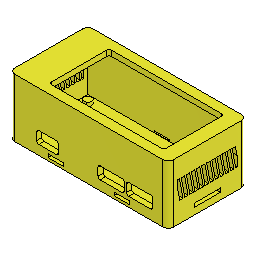
cubiea7z (Autodesk Fusion 360 design; units mm, degrees)
part number: 2026-06-29-06-27-47-318
Autodesk Fusion 360 part; units mm, degrees
sketch "Sketch1" plane through (0, 0, 0) normal (0, 0, 1) x (1, 0, 0)
  line L0 (0, 0) -> (67.4, 0)
  line L1 (67.4, 0) -> (67.4, -30.75)
  line L2 (67.4, -30.75) -> (0, -30.75)
  line L3 (0, -30.75) -> (0, 0)
  line L4 (69.9, -33.25) -> (-2.5, -33.25)
  line L5 (-2.5, -33.25) -> (-2.5, 2.5)
  line L6 (-2.5, 2.5) -> (69.9, 2.5)
  line L7 (69.9, 2.5) -> (69.9, -33.25)
  dimension "d1" = 30.75
  dimension "d2" = 67.4
  dimension "d3" = -2.5
  constraint horizontal L0
  constraint vertical L1
  constraint horizontal L2
  constraint vertical L3
  constraint coincident L0.start L3.end
  measures "d1" distance of L0.start L2.end
  measures "d2" distance of L0.start L0.end
extrude "Extrude1" add sketch "Sketch1" against normal blind 2.5 contours L0 L1 L2 L3 | L4 L5 L6 L7 makes body 1
sketch "Sketch2" plane through (0, 0, 0) normal (0, 0, 1) x (1, 0, 0)
  line L0 (67.4, -30.75) -> (0, -30.75)
  line L1 (67.4, 0) -> (67.4, -30.75)
  line L2 (0, 0) -> (67.4, 0)
  line L3 (67.4, -30.75) -> (65.4, -30.75)
  line L4 (65.4, -30.75) -> (65.4, -23.75)
  line L5 (65.4, -23.75) -> (67.4, -23.75)
  line L6 (67.4, -23.75) -> (67.4, -30.75)
  line L7 (67.4, 0) -> (65.4, 0)
  line L8 (65.4, 0) -> (65.4, -5)
  line L9 (65.4, -5) -> (67.4, -5)
  line L10 (67.4, -5) -> (67.4, 0)
  line L11 (0, -30.75) -> (0, 0)
  line L12 (0, 0) -> (2, 0)
  line L13 (2, 0) -> (2, -30.75)
  line L14 (2, -30.75) -> (0, -30.75)
  line L15 (0, -30.75) -> (0, 0)
  line L16 (67.4, 0) -> (63.4, 0)
  line L17 (63.4, 0) -> (63.4, -5)
  line L18 (63.4, -5) -> (67.4, -5)
  line L19 (67.4, -5) -> (67.4, 0)
  line L20 (67.4, -30.75) -> (63.4, -30.75)
  line L21 (63.4, -30.75) -> (63.4, -23.75)
  line L22 (63.4, -23.75) -> (67.4, -23.75)
  line L23 (67.4, -23.75) -> (67.4, -30.75)
  dimension "d6" = 2
  dimension "d7" = 7
  dimension "d8" = 2
  dimension "d9" = 5
  dimension "d10" = 2
  dimension "d11" = 4
  dimension "d12" = 5
  dimension "d13" = 4
  dimension "d14" = 7
  constraint horizontal L3
  constraint vertical L4
  constraint horizontal L5
  constraint vertical L6
  constraint coincident L0.start L1.end
  constraint horizontal L7
  constraint vertical L8
  constraint horizontal L9
  constraint vertical L10
  constraint coincident L1.start L2.end
  constraint horizontal L12
  constraint vertical L13
  constraint horizontal L14
  constraint vertical L15
  constraint coincident L2.start L11.end
  constraint horizontal L16
  constraint vertical L17
  constraint horizontal L18
  constraint vertical L19
  constraint horizontal L20
  constraint vertical L21
  constraint horizontal L22
  constraint vertical L23
  measures "d6" distance of L0.start L3.end
  measures "d7" distance of L0.start L5.end
  measures "d8" distance of L1.start L7.end
  measures "d9" distance of L1.start L9.end
  measures "d10" distance of L2.start L12.end
  measures "d11" distance of L1.start L16.end
  measures "d12" distance of L1.start L9.end
  measures "d13" distance of L0.start L20.end
  measures "d14" distance of L0.start L5.end
extrude "Extrude2" add sketch "Sketch2" along normal blind 1.2 contours L0 L4 L20 L21 L22 | L0 L2 L11 L12 L13 L14 L15 | L2 L8 L16 L17 L18 bodies 1
extrude "Extrude3" add sketch "Sketch2" along normal blind 3 contours L0 L1 L3 L4 L5 L6 L20 L22 L23 | L1 L2 L7 L8 L9 L10 L16 L18 L19 bodies 1
extrude "Extrude4" add sketch "Sketch1" along normal blind 24.1 bodies 1
ref_plane "WorkPlane1" through (34.7, -15.375, 19.4) normal (0, 0, 1) x (1, 0, 0)
sketch "USB-HDMI" plane through (0, -33.25, 0) normal (0, -1, 0) x (1, 0, 0)
  line L0 (-2.5, 24.1) -> (-2.5, -2.5)
  line L1 (-2.5, -2.5) -> (69.9, -2.5)
  line L2 (69.9, -2.5) -> (69.9, 24.1)
  line L3 (69.9, 24.1) -> (-2.5, 24.1)
  line L4 (67.4, 0) -> (63.4, 0)
  line L5 (63.4, 0) -> (2, 0)
  line L6 (2, 0) -> (63.4, 0)
  line L7 (63.4, 0) -> (67.4, 0)
  line L8 (0, 1.2) -> (0, 24.1)
  line L9 (0, 24.1) -> (0, 1.2)
  line L10 (67.4, 3) -> (67.4, 0)
  line L11 (67.4, 0) -> (67.4, 3)
  line L12 (67.4, 3) -> (67.4, 24.1)
  line L13 (67.4, 24.1) -> (67.4, 3)
  line L14 (5, 0) -> (5, 17) construction
  line L15 (5, 17) -> (29, 17) construction
  line L16 (29.5, 14.25) -> (4.5, 14.25)
  line L17 (4.5, 14.25) -> (4.5, 19.75)
  line L18 (4.5, 19.75) -> (29.5, 19.75)
  line L19 (29.5, 19.75) -> (29.5, 14.25)
  line L20 (29.5, 14.25) -> (4.5, 19.75) construction
  line L21 (4.5, 14.25) -> (29.5, 19.75) construction
  line L22 (5, 17) -> (48, 17) construction
  line L23 (48, 17) -> (57, 17) construction
  line L24 (57.5, 14.25) -> (47.5, 14.25)
  line L25 (47.5, 14.25) -> (47.5, 19.75)
  line L26 (47.5, 19.75) -> (57.5, 19.75)
  line L27 (57.5, 19.75) -> (57.5, 14.25)
  line L28 (57.5, 14.25) -> (47.5, 19.75) construction
  line L29 (47.5, 14.25) -> (57.5, 19.75) construction
  line L30 (17, 19.75) -> (17, 14.25) construction
  line L31 (17.5, 14.25) -> (16.5, 14.25)
  line L32 (16.5, 14.25) -> (16.5, 19.75)
  line L33 (16.5, 19.75) -> (17.5, 19.75)
  line L34 (17.5, 19.75) -> (17.5, 14.25)
  line L35 (17.5, 14.25) -> (16.5, 19.75) construction
  line L36 (16.5, 14.25) -> (17.5, 19.75) construction
  point P0 (17, 17)
  point P1 (52.5, 17)
  point P2 (17, 17)
  dimension "d21" = 17
  dimension "d22" = 5
  dimension "d23" = 24
  dimension "d24" = 5.5
  dimension "d25" = 25
  dimension "d26" = 43
  dimension "d27" = 9
  dimension "d28" = 10
  dimension "d29" = 5.5
  dimension "d34" = 1
  constraint perpendicular L6 L14
  constraint perpendicular L14 L15
  constraint horizontal L16
  constraint perpendicular L16 L17
  constraint parallel L16 L18
  constraint parallel L17 L19
  constraint coincident L20 P2
  constraint coincident L21 P2
  constraint midpoint L15 P2
  constraint perpendicular L14 L22
  constraint parallel L22 L23
  constraint horizontal L24
  constraint perpendicular L24 L25
  constraint parallel L24 L26
  constraint parallel L25 L27
  constraint coincident L28 P1
  constraint coincident L29 P1
  constraint midpoint L23 P1
  constraint midpoint L18 L30.start
  constraint midpoint L16 L30.end
  constraint horizontal L31
  constraint perpendicular L31 L32
  constraint parallel L31 L33
  constraint parallel L32 L34
  constraint coincident L35 P2
  constraint coincident L36 P2
  constraint coincident P2 P0
  measures "d21" distance of L14.start L14.end
  measures "d22" distance of L9 L14
  measures "d23" distance of L14.end L15.end
  measures "d24" distance of L16.end L17.end
  measures "d25" distance of L16.start L16.end
  measures "d26" distance of L14.end L22.end
  measures "d27" distance of L22.end L23.end
  measures "d28" distance of L25.end L26.end
  measures "d29" distance of L24.end L25.end
  measures "d34" distance of L32.end L33.end
extrude "Extrude5" cut sketch "USB-HDMI" against normal blind 2.5 contours L16 L18 L19 L34 | L16 L17 L18 L32 | L24 L25 L26 L27 bodies 1
fillet "Fillet1" radius 1 8 edges at (4.5, -32, 19.75) (4.5, -32, 14.25) (29.5, -32, 19.75) (29.5, -32, 14.25) (57.5, -32, 14.25) (57.5, -32, 19.75) (47.5, -32, 19.75) (47.5, -32, 14.25) on bodies 1
fillet "Fillet2" radius 1 4 edges at (17.5, -32, 19.75) (17.5, -32, 14.25) (16.5, -32, 19.75) (16.5, -32, 14.25) on bodies 1
sketch "SD-Cam" plane through (-2.5, 0, 0) normal (-1, 0, 0) x (0, -1, 0)
  line L0 (-2.5, 24.1) -> (-2.5, -2.5)
  line L1 (-2.5, -2.5) -> (33.25, -2.5)
  line L2 (33.25, -2.5) -> (33.25, 24.1)
  line L3 (33.25, 24.1) -> (-2.5, 24.1)
  line L4 (-3.075, 19.4) -> (33.825, 19.4)
  line L5 (15.375, 19.4) -> (9.375, 19.4)
  line L6 (9.375, 19.4) -> (9.375, 21.05)
  line L7 (9.375, 21.05) -> (15.375, 21.05)
  line L8 (15.375, 21.05) -> (15.375, 19.4)
  line L9 (15.375, 19.4) -> (21.375, 19.4)
  line L10 (21.375, 19.4) -> (21.375, 21.05)
  line L11 (21.375, 21.05) -> (15.375, 21.05)
  line L12 (15.375, 21.05) -> (15.375, 19.4)
  dimension "d38" = 6
  dimension "d39" = 1.65
  dimension "d40" = 1.65
  constraint horizontal L5
  constraint vertical L6
  constraint horizontal L7
  constraint vertical L8
  constraint midpoint L4 L5.start
  constraint horizontal L9
  constraint vertical L10
  constraint horizontal L11
  constraint vertical L12
  measures "d38" distance of L5.start L5.end
  measures "d39" distance of L5.start L7.end
  measures "d40" distance of L5.start L7.end
extrude "Extrude6" cut sketch "SD-Cam" against normal blind 2.5 contours L4 L5 L6 L7 L8 L12 | L4 L8 L9 L10 L11 L12 bodies 1
fillet "Fillet3" radius 0.3 4 edges at (-1.25, -9.375, 21.05) (-1.25, -9.375, 19.4) (-1.25, -21.375, 21.05) (-1.25, -21.375, 19.4) on bodies 1
extrude "Extrude7" cut sketch "SD-Cam" against normal blind 72.4 contours L4 L5 L6 L7 L8 L12 | L4 L8 L9 L10 L11 L12 bodies 1
sketch "Antenne" plane through (69.9, 0, 0) normal (1, 0, 0) x (0, 1, 0)
  line L0 (-21.375, 19.4) -> (-21.375, 21.05)
  line L1 (-21.375, 21.05) -> (-9.375, 21.05)
  line L2 (-9.375, 21.05) -> (-9.375, 19.4)
  line L3 (-9.375, 19.4) -> (-21.375, 19.4)
  line L4 (-33.25, 24.1) -> (-33.25, -2.5)
  line L5 (-33.25, -2.5) -> (2.5, -2.5)
  line L6 (2.5, -2.5) -> (2.5, 24.1)
  line L7 (2.5, 24.1) -> (-33.25, 24.1)
  line L8 (3.075, 19.4) -> (-33.825, 19.4)
  line L9 (3.075, 18.4) -> (-33.825, 18.4) construction
  line L10 (-15.375, 18.4) -> (-17.375, 18.4)
  line L11 (-17.375, 18.4) -> (-17.375, 15.4)
  line L12 (-17.375, 15.4) -> (-15.375, 15.4)
  line L13 (-15.375, 15.4) -> (-15.375, 18.4)
  line L14 (-15.375, 18.4) -> (-13.375, 18.4)
  line L15 (-13.375, 18.4) -> (-13.375, 15.4)
  line L16 (-13.375, 15.4) -> (-15.375, 15.4)
  line L17 (-15.375, 15.4) -> (-15.375, 18.4)
  dimension "d47" = -1
  dimension "d48" = 2
  dimension "d49" = 3
  dimension "d50" = 3
  constraint horizontal L10
  constraint vertical L11
  constraint horizontal L12
  constraint vertical L13
  constraint midpoint L9 L10.start
  constraint horizontal L14
  constraint vertical L15
  constraint horizontal L16
  constraint vertical L17
  measures "d48" distance of L10.start L10.end
  measures "d49" distance of L10.start L12.end
  measures "d50" distance of L10.start L12.end
extrude "Extrude8" cut sketch "Antenne" against normal blind 2.5 contours L10 L11 L12 L13 L17 | L13 L14 L15 L16 L17 bodies 1
fillet "Fillet4" radius 0.3 4 edges at (68.65, -21.375, 21.05) (68.65, -9.375, 21.05) (68.65, -9.375, 19.4) (68.65, -21.375, 19.4) on bodies 1
fillet "Fillet5" radius 0.5 4 edges at (68.65, -17.375, 18.4) (68.65, -17.375, 15.4) (68.65, -13.375, 18.4) (68.65, -13.375, 15.4) on bodies 1
sketch "Skjermhull" plane through (0, 0, -2.5) normal (0, 0, -1) x (1, 0, 0)
  line L0 (-2.5, -2.5) -> (69.9, -2.5)
  line L1 (69.9, -2.5) -> (69.9, 33.25)
  line L2 (69.9, 33.25) -> (-2.5, 33.25)
  line L3 (-2.5, 33.25) -> (-2.5, -2.5)
  line L4 (0, 21.375) -> (0, 9.375)
  line L5 (0, 9.375) -> (0, 21.375)
  line L6 (0, 30.75) -> (0, 0)
  line L7 (0, 0) -> (0, 30.75)
  line L8 (67.4, 17.375) -> (67.4, 16.875)
  line L9 (67.4, 16.875) -> (67.4, 13.875)
  line L10 (67.4, 13.875) -> (67.4, 13.375)
  line L11 (67.4, 13.875) -> (67.4, 13.375)
  line L12 (67.4, 13.875) -> (67.4, 16.875)
  line L13 (67.4, 17.375) -> (67.4, 16.875)
  line L14 (67.4, 21.375) -> (67.4, 21.075)
  line L15 (67.4, 21.075) -> (67.4, 9.675)
  line L16 (67.4, 9.675) -> (67.4, 9.375)
  line L17 (67.4, 9.675) -> (67.4, 9.375)
  line L18 (67.4, 9.675) -> (67.4, 21.075)
  line L19 (67.4, 21.375) -> (67.4, 21.075)
  line L20 (67.4, 0) -> (67.4, 5)
  line L21 (67.4, 5) -> (67.4, 23.75)
  line L22 (67.4, 23.75) -> (67.4, 30.75)
  line L23 (67.4, 30.75) -> (67.4, 0)
  line L24 (65.4, 0) -> (67.4, 0)
  line L25 (67.4, 0) -> (0, 0)
  line L26 (0, 0) -> (2, 0)
  line L27 (2, 0) -> (63.4, 0)
  line L28 (63.4, 0) -> (65.4, 0)
  line L29 (15.5, 30.75) -> (16.5, 30.75)
  line L30 (15.5, 30.75) -> (5.5, 30.75)
  line L31 (4.5, 30.75) -> (5.5, 30.75)
  line L32 (4.5, 30.75) -> (5.5, 30.75)
  line L33 (5.5, 30.75) -> (15.5, 30.75)
  line L34 (15.5, 30.75) -> (16.5, 30.75)
  line L35 (17.5, 30.75) -> (18.5, 30.75)
  line L36 (18.5, 30.75) -> (28.5, 30.75)
  line L37 (28.5, 30.75) -> (29.5, 30.75)
  line L38 (28.5, 30.75) -> (29.5, 30.75)
  line L39 (28.5, 30.75) -> (18.5, 30.75)
  line L40 (17.5, 30.75) -> (18.5, 30.75)
  line L41 (47.5, 30.75) -> (48.5, 30.75)
  line L42 (48.5, 30.75) -> (56.5, 30.75)
  line L43 (56.5, 30.75) -> (57.5, 30.75)
  line L44 (56.5, 30.75) -> (57.5, 30.75)
  line L45 (56.5, 30.75) -> (48.5, 30.75)
  line L46 (47.5, 30.75) -> (48.5, 30.75)
  line L47 (67.4, 30.75) -> (65.4, 30.75)
  line L48 (65.4, 30.75) -> (63.4, 30.75)
  line L49 (63.4, 30.75) -> (2, 30.75)
  line L50 (2, 30.75) -> (0, 30.75)
  line L51 (0, 30.75) -> (67.4, 30.75)
  line L52 (3.7, 29.05) -> (56, 29.05)
  line L53 (56, 29.05) -> (56, 1.7)
  line L54 (56, 1.7) -> (3.7, 1.7)
  line L55 (3.7, 1.7) -> (3.7, 29.05)
  dimension "d57" = 3.7
  dimension "d58" = 1.7
  dimension "d59" = 1.7
  dimension "d60" = 56
  constraint horizontal L52
  constraint vertical L53
  constraint horizontal L54
  constraint vertical L55
  measures "d57" distance of L5 L55
  measures "d58" distance of L49 L52
  measures "d59" distance of L25 L54
  measures "d60" distance of L6 L53
extrude "Extrude9" cut sketch "Skjermhull" against normal blind 2.5 contours L52 L53 L54 L55 bodies 1
fillet "Fillet6" radius 1 4 edges at (3.7, -29.05, -1.25) (56, -29.05, -1.25) (56, -1.7, -1.25) (3.7, -1.7, -1.25) on bodies 1
sketch "Sketch7" plane through (69.9, 0, 0) normal (1, 0, 0) x (0, 1, 0)
  line L0 (-17.375, 15.9) -> (-17.375, 17.9)
  arc A0 (-16.875, 18.4) -> (-17.375, 17.9) centre (-16.875, 17.9) ccw
  line L1 (-16.875, 18.4) -> (-13.875, 18.4)
  arc A1 (-13.375, 17.9) -> (-13.875, 18.4) centre (-13.875, 17.9) ccw
  line L2 (-13.375, 17.9) -> (-13.375, 15.9)
  arc A2 (-13.875, 15.4) -> (-13.375, 15.9) centre (-13.875, 15.9) ccw
  line L3 (-13.875, 15.4) -> (-16.875, 15.4)
  arc A3 (-17.375, 15.9) -> (-16.875, 15.4) centre (-16.875, 15.9) ccw
  line L4 (-21.375, 19.7) -> (-21.375, 20.75)
  arc A4 (-21.075, 21.05) -> (-21.375, 20.75) centre (-21.075, 20.75) ccw
  line L5 (-21.075, 21.05) -> (-9.675, 21.05)
  arc A5 (-9.375, 20.75) -> (-9.675, 21.05) centre (-9.675, 20.75) ccw
  line L6 (-9.375, 20.75) -> (-9.375, 19.7)
  arc A6 (-9.675, 19.4) -> (-9.375, 19.7) centre (-9.675, 19.7) ccw
  line L7 (-9.675, 19.4) -> (-21.075, 19.4)
  arc A7 (-21.375, 19.7) -> (-21.075, 19.4) centre (-21.075, 19.7) ccw
  line L8 (-33.25, 24.1) -> (-33.25, -2.5)
  line L9 (-33.25, -2.5) -> (2.5, -2.5)
  line L10 (2.5, -2.5) -> (2.5, 24.1)
  line L11 (2.5, 24.1) -> (-33.25, 24.1)
  line L12 (-28.875, 14.9) -> (-1.875, 14.9)
  line L13 (-1.875, 14.9) -> (-1.875, 6.4)
  line L14 (-1.875, 6.4) -> (-28.875, 6.4)
  line L15 (-28.875, 6.4) -> (-28.875, 14.9)
  line L16 (-15.375, 15.4) -> (-15.375, 14.4) construction
  line L17 (-29.6028, 6.4) -> (-28.0015, 14.9)
  line L18 (-28.0015, 14.9) -> (-26.5, 14.9)
  line L19 (-26.5, 14.9) -> (-28.1013, 6.4)
  line L20 (-28.1013, 6.4) -> (-29.6028, 6.4)
  line L21 (-24.1818, 14.9) -> (-25.7831, 6.4)
  line L22 (-25.6833, 14.9) -> (-24.1818, 14.9)
  line L23 (-27.2846, 6.4) -> (-25.6833, 14.9)
  line L24 (-25.7831, 6.4) -> (-27.2846, 6.4)
  line L25 (-21.8636, 14.9) -> (-23.4649, 6.4)
  line L26 (-23.3651, 14.9) -> (-21.8636, 14.9)
  line L27 (-24.9664, 6.4) -> (-23.3651, 14.9)
  line L28 (-23.4649, 6.4) -> (-24.9664, 6.4)
  line L29 (-19.5455, 14.9) -> (-21.1467, 6.4)
  line L30 (-21.0469, 14.9) -> (-19.5455, 14.9)
  line L31 (-22.6482, 6.4) -> (-21.0469, 14.9)
  line L32 (-21.1467, 6.4) -> (-22.6482, 6.4)
  line L33 (-17.2273, 14.9) -> (-18.8285, 6.4)
  line L34 (-18.7288, 14.9) -> (-17.2273, 14.9)
  line L35 (-20.33, 6.4) -> (-18.7288, 14.9)
  line L36 (-18.8285, 6.4) -> (-20.33, 6.4)
  line L37 (-14.9091, 14.9) -> (-16.5104, 6.4)
  line L38 (-16.4106, 14.9) -> (-14.9091, 14.9)
  line L39 (-18.0118, 6.4) -> (-16.4106, 14.9)
  line L40 (-16.5104, 6.4) -> (-18.0118, 6.4)
  line L41 (-12.5909, 14.9) -> (-14.1922, 6.4)
  line L42 (-14.0924, 14.9) -> (-12.5909, 14.9)
  line L43 (-15.6937, 6.4) -> (-14.0924, 14.9)
  line L44 (-14.1922, 6.4) -> (-15.6937, 6.4)
  line L45 (-10.2727, 14.9) -> (-11.874, 6.4)
  line L46 (-11.7742, 14.9) -> (-10.2727, 14.9)
  line L47 (-13.3755, 6.4) -> (-11.7742, 14.9)
  line L48 (-11.874, 6.4) -> (-13.3755, 6.4)
  line L49 (-7.9545, 14.9) -> (-9.5558, 6.4)
  line L50 (-9.456, 14.9) -> (-7.9545, 14.9)
  line L51 (-11.0573, 6.4) -> (-9.456, 14.9)
  line L52 (-9.5558, 6.4) -> (-11.0573, 6.4)
  line L53 (-5.6364, 14.9) -> (-7.2376, 6.4)
  line L54 (-7.1379, 14.9) -> (-5.6364, 14.9)
  line L55 (-8.7391, 6.4) -> (-7.1379, 14.9)
  line L56 (-7.2376, 6.4) -> (-8.7391, 6.4)
  line L57 (-3.3182, 14.9) -> (-4.9194, 6.4)
  line L58 (-4.8197, 14.9) -> (-3.3182, 14.9)
  line L59 (-6.4209, 6.4) -> (-4.8197, 14.9)
  line L60 (-4.9194, 6.4) -> (-6.4209, 6.4)
  line L61 (-1, 14.9) -> (-2.6013, 6.4)
  line L62 (-2.5015, 14.9) -> (-1, 14.9)
  line L63 (-4.1028, 6.4) -> (-2.5015, 14.9)
  line L64 (-2.6013, 6.4) -> (-4.1028, 6.4)
  dimension "d65" = 0.5
  dimension "d66" = 8.5
  dimension "d67" = 27
  dimension "d70" = 25.5
  dimension "d71" = 0
  constraint horizontal L12
  constraint vertical L13
  constraint horizontal L14
  constraint vertical L15
  constraint midpoint L3 L16.start
  constraint perpendicular L12 L16
  constraint midpoint L12 L16
  constraint coincident L14 L17.start
  constraint coincident L12 L17.end
  constraint coincident L12 L18.end
  constraint coincident L14 L19.end
  constraint parallel L17 L19
  measures "d65" distance of L3 L12
  measures "d66" distance of L12 L14
  measures "d67" distance of L13 L15
extrude "Extrude10" cut sketch "Sketch7" against normal blind 72.4 contours L12 L14 L15 L17 L18 L19 L20 | L12 L14 L21 L22 L23 L24 | L12 L14 L25 L26 L27 L28 | L12 L14 L29 L30 L31 L32 | L12 L14 L33 L34 L35 L36 | L12 L14 L37 L38 L39 L40 | L12 L14 L41 L42 L43 L44 | L12 L14 L45 L46 L47 L48 | L12 L14 L49 L50 L51 L52 | L12 L14 L53 L54 L55 L56 | L12 L14 L57 L58 L59 L60 | L12 L13 L14 L61 L62 L63 L64 bodies 1
sketch "Festehull" plane through (0, 2.5, 0) normal (0, 1, 0) x (-1, 0, 0)
  line L0 (-69.9, 24.1) -> (-69.9, -2.5)
  line L1 (-69.9, -2.5) -> (2.5, -2.5)
  line L2 (2.5, -2.5) -> (2.5, 24.1)
  line L3 (2.5, 24.1) -> (-69.9, 24.1)
  line L4 (-33.7, 24.1) -> (-33.7, 21.6) construction
  line L5 (-33.7, 21.6) -> (-30.2, 21.6)
  line L6 (-30.2, 21.6) -> (-30.2, 22.85)
  line L7 (-30.2, 22.85) -> (-33.7, 22.85)
  line L8 (-33.7, 21.6) -> (-37.2, 21.6)
  line L9 (-37.2, 21.6) -> (-37.2, 22.85)
  line L10 (-37.2, 22.85) -> (-33.7, 22.85)
  line L11 (-18.7, 21.6) -> (-22.2, 21.6)
  line L12 (-22.2, 21.6) -> (-22.2, 22.85)
  line L13 (-22.2, 22.85) -> (-18.7, 22.85)
  line L14 (-15.2, 22.85) -> (-18.7, 22.85)
  line L15 (-18.7, 21.6) -> (-15.2, 21.6)
  line L16 (-15.2, 21.6) -> (-15.2, 22.85)
  line L17 (-48.7, 21.6) -> (-52.2, 21.6)
  line L18 (-48.7, 21.6) -> (-45.2, 21.6)
  line L19 (-45.2, 21.6) -> (-45.2, 22.85)
  line L20 (-45.2, 22.85) -> (-48.7, 22.85)
  line L21 (-52.2, 22.85) -> (-48.7, 22.85)
  line L22 (-52.2, 21.6) -> (-52.2, 22.85)
  dimension "d74" = 2.5
  dimension "d75" = 3.5
  dimension "d76" = 1.25
  dimension "d77" = 1.25
  dimension "d80" = 15
  dimension "d81" = 0
  dimension "d84" = -15
  dimension "d85" = 0
  constraint midpoint L3 L4.start
  constraint perpendicular L3 L4
  constraint horizontal L5
  constraint vertical L6
  constraint horizontal L7
  constraint horizontal L8
  constraint vertical L9
  constraint horizontal L10
  measures "d74" distance of L4.start L4.end
  measures "d75" distance of L4.end L5.end
  measures "d76" distance of L4.end L7.end
  measures "d77" distance of L4.end L7.end
extrude "Extrude11" cut sketch "Festehull" along normal up to surface (2.5 mm away) from surface at -35.75 contours L11 L12 L13 L14 L15 L16 | L17 L18 L19 L20 L21 L22 bodies 1
extrude "Extrude12" cut sketch "Festehull" against normal blind 2.5 contours L5 L6 L7 L8 L9 L10 bodies 1
sketch "Bunnplate" plane through (0, 0, 24.1) normal (0, 0, 1) x (-1, 0, 0)
  line L0 (-67.4, 30.75) -> (0, 30.75)
  line L1 (0, 30.75) -> (0, 0)
  line L2 (0, 0) -> (-67.4, 0)
  line L3 (-67.4, 0) -> (-67.4, 30.75)
  line L4 (-69.9, -2.5) -> (2.5, -2.5)
  line L5 (2.5, -2.5) -> (2.5, 33.25)
  line L6 (2.5, 33.25) -> (-69.9, 33.25)
  line L7 (-69.9, 33.25) -> (-69.9, -2.5)
  line L8 (-67.4, 0) -> (-67.4, 30.75)
  line L9 (-67.4, 30.75) -> (0, 30.75)
  line L10 (0, 30.75) -> (0, 0)
  line L11 (0, 0) -> (-67.4, 0)
  line L12 (-0.2, 0.2) -> (-67.2, 0.2)
  line L13 (-67.2, 0.2) -> (-67.2, 30.55)
  line L14 (-67.2, 30.55) -> (-0.2, 30.55)
  line L15 (-0.2, 30.55) -> (-0.2, 0.2)
  dimension "d91" = 0.2
extrude "Extrude13" add sketch "Bunnplate" against normal blind 2.5 separate body contours L12 L13 L14 L15 makes body 2
extrude "Extrude14" add sketch "Festehull" against normal blind 2.7 contours L5 L6 L7 L8 L9 L10 bodies 2
extrude "Extrude15" add sketch "Festehull" along normal blind 3 from surface at -35.75 contours L11 L12 L13 L14 L15 L16 | L17 L18 L19 L20 L21 L22 bodies 2
move_face "OffsetFaces1" offset -0.1 6 faces at (45.2, -32.35, 22.0167) (52.2, -32.35, 22.0167) (22.2, -32.35, 22.0167) (15.2, -32.35, 22.0167) (30.2, 1.6, 22.0167) (37.2, 1.6, 22.0167) on bodies 2
move_face "OffsetFaces2" offset -0.1 3 faces at (32.5667, 0.7, 22.85) (17.5667, -31.45, 22.85) (47.5667, -31.45, 22.85) on bodies 2
move_face "OffsetFaces3" offset -1 3 faces at (34.8333, 2.5, 22.3667) (49.8333, -33.25, 22.3667) (17.5667, -33.25, 22.3667) on bodies 2
chamfer "Chamfer1" distance 0.5 angle 45 3 edges at (33.7, 1.5, 22.75) (48.7, -32.25, 22.75) (18.7, -32.25, 22.75) on bodies 2
fillet "Fillet7" radius 2.5 4 edges at (-2.5, -33.25, 10.8) (-2.5, 2.5, 10.8) (69.9, 2.5, 10.8) (69.9, -33.25, 10.8) on bodies 1
move_face "OffsetFaces4" offset -0.2 3 faces at (34.8667, 1.6667, 21.6) (47.5333, -32.4167, 21.6) (17.5333, -32.4167, 21.6) on bodies 1
move_face "OffsetFaces5" offset -0.1 4 faces at (31.8667, 0, 7.1333) (0, -4.2311, 20.0167) (31.3474, -30.75, 4.7534) (67.4, -14.3141, 2.1333) on bodies 1
move_face "OffsetFaces6" offset -0.1 1 faces at (52.1333, -10.3167, 21.6) on bodies 2
sketch "Sketch10" plane through (0, 0, 21.7) normal (0, 0, -1) x (1, 0, 0)
  line L0 (45.3, 30.55) -> (22.1, 30.55)
  line L1 (22.1, 30.55) -> (22.1, 32.25)
  line L2 (22.1, 32.25) -> (15.3, 32.25)
  line L3 (15.3, 32.25) -> (15.3, 30.55)
  line L4 (15.3, 30.55) -> (0.2, 30.55)
  line L5 (0.2, 30.55) -> (0.2, 0.2)
  line L6 (0.2, 0.2) -> (30.3, 0.2)
  line L7 (30.3, 0.2) -> (30.3, -1.5)
  line L8 (30.3, -1.5) -> (37.1, -1.5)
  line L9 (37.1, -1.5) -> (37.1, 0.2)
  line L10 (37.1, 0.2) -> (67.2, 0.2)
  line L11 (67.2, 0.2) -> (67.2, 30.55)
  line L12 (67.2, 30.55) -> (52.1, 30.55)
  line L13 (52.1, 30.55) -> (52.1, 32.25)
  line L14 (52.1, 32.25) -> (45.3, 32.25)
  line L15 (45.3, 32.25) -> (45.3, 30.55)
  line L16 (67.2, 0.2) -> (0.2, 0.2)
  line L17 (0.2, 0.2) -> (0.2, 30.55)
  line L18 (0.2, 30.55) -> (67.2, 30.55)
  line L19 (67.2, 30.55) -> (67.2, 0.2)
  line L20 (67.2, 5.2) -> (0.2, 5.2)
  line L21 (0.2, 5.2) -> (0.2, 25.55)
  line L22 (0.2, 25.55) -> (67.2, 25.55)
  line L23 (67.2, 25.55) -> (67.2, 5.2)
  circle A0 centre (63.7, 3.7) radius 1.75
  circle A1 centre (63.7, 27.05) radius 1.75
  circle A2 centre (5.7, 27.05) radius 1.75
  circle A3 centre (5.7, 3.7) radius 1.75
  dimension "d108" = 5
  dimension "d109" = 5
  dimension "d114" = 3.5
  dimension "d115" = 3.5
  dimension "d116" = 3.5
  dimension "d117" = 3.5
  dimension "d118" = 3.5
  dimension "d119" = 3.5
  dimension "d120" = 3.5
  dimension "d121" = 3.5
  dimension "d122" = 3.5
  dimension "d123" = 3.5
  dimension "d124" = 61.5
  dimension "d125" = 61.5
  constraint horizontal L16
  constraint vertical L17
  constraint horizontal L18
  constraint vertical L19
  constraint coincident L4.end L5.start
  constraint coincident L10.end L11.start
  constraint horizontal L20
  constraint vertical L21
  constraint horizontal L22
  constraint vertical L23
  constraint coincident L17 L21.end
  constraint coincident L19 L20.start
  measures "d108" distance of L16 L20
  measures "d109" distance of L18 L22
  measures "d114" diameter of A0
  measures "d115" diameter of A1
  measures "d116" distance of L16 A0.centre
  measures "d117" distance of L19 A0.centre
  measures "d118" distance of L18 A1.centre
  measures "d119" distance of L19 A1.centre
  measures "d120" diameter of A2
  measures "d121" diameter of A3
  measures "d122" distance of L16 A3.centre
  measures "d123" distance of L18 A2.centre
  measures "d124" distance of L19 A3.centre
  measures "d125" distance of L19 A2.centre
extrude "Extrude16" cut sketch "Sketch10" against normal blind 1.2 contours L5 L11 L17 L19 L20 L21 L22 L23 A0 A1 A2 A3 | L22 A1 | L22 A2 | L20 A0 | L20 A3 picked at (63.9303, 25.514) picked at (5.9303, 25.514) picked at (63.4739, 5.2981) picked at (5.6213, 5.3499) bodies 2
extrude "Extrude17" cut sketch "Sketch10" against normal blind 0.2 contours L0 L4 L5 L11 L12 L17 L18 L19 L22 A1 A2 | L5 L6 L10 L11 L16 L17 L19 L20 A0 A3 | L22 A1 | L22 A2 | L20 A0 | L20 A3 picked at (63.97, 27.9375) picked at (5.5745, 26.6197) picked at (64.1261, 3.9972) picked at (5.4913, 4.1553) bodies 2
extrude "Extrude18" add sketch "Sketch10" along normal blind 1.4 and the other way blind 1 contours L22 A1 | L22 A2 | L20 A0 | L20 A3 picked at (63.97, 27.9375) picked at (5.5745, 26.6197) picked at (64.1261, 3.9972) picked at (5.4913, 4.1553) bodies 2
equation "d19 = 21.1 mm + 0.5 mm + 2.5 mm"
equation "d26 = 48 mm - 5 mm"
